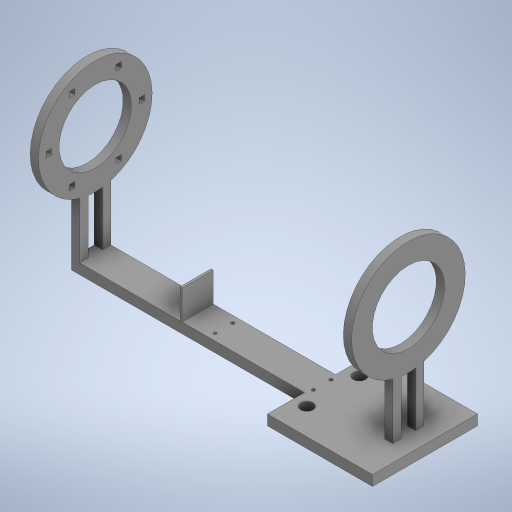
# Autodesk Inventor part: base
Saved by Autodesk Inventor 2023 (Build 270158000, 158)
## iProperties
Created: 2022-11-02
Part Number: base
Material: Generic
Document SubType Name: Modeling
Designer: Admin
Density: 1 g/cm^3
Appearance: Default
Author: Admin
Autodesk Inventor part; units mm, degrees
ref_plane "YZ Plane" through (0, 0, 0) normal (1, 0, 0) x (0, 1, 0)
ref_plane "XZ Plane" through (0, 0, 0) normal (0, 1, 0) x (-1, 0, 0)
ref_plane "XY Plane" through (0, 0, 0) normal (0, 0, 1) x (1, 0, 0)
sketch "Sketch1" plane through (0, 0, 0) normal (1, 0, 0) x (0, 1, 0)
  line L0 (38.9711, 22.5) -> (38.9711, -22.5)
  line L1 (38.9711, -22.5) -> (0, -45)
  line L2 (0, -45) -> (-38.9711, -22.5)
  line L3 (-38.9711, -22.5) -> (-38.9711, 22.5)
  line L4 (-38.9711, 22.5) -> (0, 45)
  line L5 (0, 45) -> (38.9711, 22.5)
  line L6 (0, 45) -> (0, -45)
  line L7 (38.9711, 0) -> (-38.9711, 0)
  circle A0 centre (38.9711, -22.5) radius 17.5
  circle A1 centre (38.9711, -22.5) radius 12.5
  circle A2 centre (38.9711, -22.5) radius 10.4
  circle A3 centre (38.9711, -22.5) radius 15
  line L8 (38.9711, -22.5) -> (62.5188, -22.5)
  line L9 (56.4711, -26.5) -> (64.4711, -26.5)
  line L10 (64.4711, -26.5) -> (64.4711, -18.5)
  line L11 (64.4711, -18.5) -> (56.4711, -18.5)
  line L12 (56.4711, -18.5) -> (56.4711, -26.5)
  line L13 (56.4711, -26.5) -> (64.4711, -18.5) construction
  line L14 (64.4711, -26.5) -> (56.4711, -18.5) construction
  circle A4 centre (38.9711, 22.5) radius 10.4
  circle A5 centre (38.9711, 22.5) radius 12.5
  circle A6 centre (0, 45) radius 10.4
  circle A7 centre (0, 45) radius 12.5
  circle A8 centre (-38.9711, 22.5) radius 10.4
  circle A9 centre (-38.9711, 22.5) radius 12.5
  circle A10 centre (-38.9711, -22.5) radius 10.4
  circle A11 centre (-38.9711, -22.5) radius 12.5
  circle A12 centre (0, -45) radius 10.4
  circle A13 centre (0, -45) radius 12.5
  line L15 (42.9711, 10.6573) -> (42.9711, -10.6573)
  line L16 (34.9711, 10.6573) -> (34.9711, -10.6573)
  line L17 (12.2561, 42.5427) -> (30.715, 31.8855)
  line L18 (8.2561, 35.6145) -> (26.715, 24.9573)
  line L19 (-30.715, 31.8855) -> (-12.2561, 42.5427)
  line L20 (-26.715, 24.9573) -> (-8.2561, 35.6145)
  line L21 (-42.9711, -10.6573) -> (-42.9711, 10.6573)
  line L22 (-34.9711, -10.6573) -> (-34.9711, 10.6573)
  line L23 (-12.2561, -42.5427) -> (-30.715, -31.8855)
  line L24 (-8.2561, -35.6145) -> (-26.715, -24.9573)
  line L25 (30.715, -31.8855) -> (12.2561, -42.5427)
  line L26 (26.715, -24.9573) -> (8.2561, -35.6145)
  line L27 (38.9711, 22.5) -> (0, 0)
  line L28 (29.9645, 17.3) -> (28.1458, 16.25)
  line L29 (-48.9711, -15) -> (-48.9711, 15)
  line L30 (-48.9711, 15) -> (-56.9711, 15)
  line L31 (-56.9711, 15) -> (-56.9711, -15)
  line L32 (-56.9711, -15) -> (-48.9711, -15)
  circle A14 centre (-38.9711, -22.5) radius 17.5
  circle A15 centre (-38.9711, 22.5) radius 17.5
  line L33 (-52.9711, -15) -> (-52.9711, 15)
  line L34 (57.8711, -25.1) -> (63.0711, -25.1)
  line L35 (63.0711, -25.1) -> (63.0711, -19.9)
  line L36 (63.0711, -19.9) -> (57.8711, -19.9)
  line L37 (57.8711, -19.9) -> (57.8711, -25.1)
  line L38 (57.8711, -25.1) -> (63.0711, -19.9) construction
  line L39 (63.0711, -25.1) -> (57.8711, -19.9) construction
  circle A16 centre (38.9711, 22.5) radius 17.5
  circle A17 centre (0, 45) radius 17.5
  circle A18 centre (-38.9711, 22.5) radius 17.5
  circle A19 centre (-38.9711, -22.5) radius 17.5
  circle A20 centre (0, -45) radius 17.5
  line L40 (0, -45) -> (30.2711, -45)
  line L41 (17.5, -49) -> (25.5, -49)
  line L42 (25.5, -49) -> (25.5, -41)
  line L43 (25.5, -41) -> (17.5, -41)
  line L44 (17.5, -41) -> (17.5, -49)
  line L45 (17.5, -49) -> (25.5, -41) construction
  line L46 (25.5, -49) -> (17.5, -41) construction
  line L47 (18.9, -47.6) -> (24.1, -47.6)
  line L48 (24.1, -47.6) -> (24.1, -42.4)
  line L49 (24.1, -42.4) -> (18.9, -42.4)
  line L50 (18.9, -42.4) -> (18.9, -47.6)
  line L51 (18.9, -47.6) -> (24.1, -42.4) construction
  line L52 (24.1, -47.6) -> (18.9, -42.4) construction
  line L53 (-38.9711, -22.5) -> (-4.25, -22.5)
  line L54 (-21.4711, -26.5) -> (-13.4711, -26.5)
  line L55 (-13.4711, -26.5) -> (-13.4711, -18.5)
  line L56 (-13.4711, -18.5) -> (-21.4711, -18.5)
  line L57 (-21.4711, -18.5) -> (-21.4711, -26.5)
  line L58 (-21.4711, -26.5) -> (-13.4711, -18.5) construction
  line L59 (-13.4711, -26.5) -> (-21.4711, -18.5) construction
  line L60 (-20.0711, -25.1) -> (-14.8711, -25.1)
  line L61 (-14.8711, -25.1) -> (-14.8711, -19.9)
  line L62 (-14.8711, -19.9) -> (-20.0711, -19.9)
  line L63 (-20.0711, -19.9) -> (-20.0711, -25.1)
  line L64 (-20.0711, -25.1) -> (-14.8711, -19.9) construction
  line L65 (-14.8711, -25.1) -> (-20.0711, -19.9) construction
  line L66 (56.4711, 26.5) -> (64.4711, 26.5)
  line L67 (64.4711, 26.5) -> (64.4711, 18.5)
  line L68 (64.4711, 18.5) -> (56.4711, 18.5)
  line L69 (56.4711, 18.5) -> (56.4711, 26.5)
  line L70 (56.4711, 26.5) -> (64.4711, 18.5) construction
  line L71 (64.4711, 26.5) -> (56.4711, 18.5) construction
  line L72 (57.8711, 25.1) -> (63.0711, 25.1)
  line L73 (63.0711, 25.1) -> (63.0711, 19.9)
  line L74 (63.0711, 19.9) -> (57.8711, 19.9)
  line L75 (57.8711, 19.9) -> (57.8711, 25.1)
  line L76 (57.8711, 25.1) -> (63.0711, 19.9) construction
  line L77 (63.0711, 25.1) -> (57.8711, 19.9) construction
  line L78 (17.5, 49) -> (25.5, 49)
  line L79 (25.5, 49) -> (25.5, 41)
  line L80 (25.5, 41) -> (17.5, 41)
  line L81 (17.5, 41) -> (17.5, 49)
  line L82 (17.5, 49) -> (25.5, 41) construction
  line L83 (25.5, 49) -> (17.5, 41) construction
  line L84 (18.9, 47.6) -> (24.1, 47.6)
  line L85 (24.1, 47.6) -> (24.1, 42.4)
  line L86 (24.1, 42.4) -> (18.9, 42.4)
  line L87 (18.9, 42.4) -> (18.9, 47.6)
  line L88 (18.9, 47.6) -> (24.1, 42.4) construction
  line L89 (24.1, 47.6) -> (18.9, 42.4) construction
  line L90 (-21.4711, 26.5) -> (-13.4711, 26.5)
  line L91 (-13.4711, 26.5) -> (-13.4711, 18.5)
  line L92 (-13.4711, 18.5) -> (-21.4711, 18.5)
  line L93 (-21.4711, 18.5) -> (-21.4711, 26.5)
  line L94 (-21.4711, 26.5) -> (-13.4711, 18.5) construction
  line L95 (-13.4711, 26.5) -> (-21.4711, 18.5) construction
  line L96 (-20.0711, 25.1) -> (-14.8711, 25.1)
  line L97 (-14.8711, 25.1) -> (-14.8711, 19.9)
  line L98 (-14.8711, 19.9) -> (-20.0711, 19.9)
  line L99 (-20.0711, 19.9) -> (-20.0711, 25.1)
  line L100 (-20.0711, 25.1) -> (-14.8711, 19.9) construction
  line L101 (-14.8711, 25.1) -> (-20.0711, 19.9) construction
  line L102 (0, 0) -> (21.5, 0)
  circle A21 centre (21.5, 0) radius 55
  circle A22 centre (21.5, 0) radius 35
  line L103 (-31.415, 0) -> (-31.415, 15)
  line L104 (-31.415, 15) -> (-85.4711, 15)
  line L105 (-85.4711, 15) -> (-85.4711, 0)
  line L106 (-31.415, 7) -> (-85.4711, 7)
  line L107 (-85.4711, 15) -> (-95.4711, 15)
  line L108 (-95.4711, 15) -> (-95.4711, -10)
  line L109 (-31.415, 0) -> (-31.415, -15)
  line L110 (-31.415, -15) -> (-85.4711, -15)
  line L111 (-85.4711, -15) -> (-85.4711, 0)
  line L112 (-31.415, -7) -> (-85.4711, -7)
  line L113 (-85.4711, -15) -> (-95.4711, -15)
  line L114 (-95.4711, -15) -> (-95.4711, -10)
  point P0 (60.4711, -22.5)
  point P1 (-42.9711, 10.6573)
  point P2 (21.5, -45)
  point P3 (-17.4711, -22.5)
  point P4 (60.4711, 22.5)
  point P5 (21.5, 45)
  point P6 (-17.4711, 22.5)
  point P7 (-31.415, -15)
  point P8 (-31.7663, 15)
  point P9 (-31.2665, 15.5144)
  point P10 (-31.2665, -15.5144)
  point P11 (-31.7663, -15)
  point P12 (-56.9711, 7)
  point P13 (-31.7663, 15)
  point P14 (-46.176, 15)
  point P15 (-56.9711, -7)
  point P16 (-33.0527, 7)
  point P17 (-33.0527, -7)
  point P18 (-28.5742, -22.7504)
  point P19 (-28.5742, 22.7504)
  point P20 (-46.176, -15)
  point P21 (-31.7663, -15)
  dimension "d45" = 110
  dimension "d8" = 35
  dimension "d9" = 45
  dimension "d10" = 25
  dimension "d11" = 20.8
  dimension "d12" = 30
  dimension "d13" = 8
  dimension "d14" = 8
  dimension "d15" = 360
  dimension "d16" = 4
  dimension "d17" = 4
  dimension "d18" = 360
  dimension "d22" = 30
  dimension "d23" = 8
  dimension "d24" = 30
  dimension "d25" = 35
  dimension "d26" = 35
  dimension "d27" = 4
  dimension "d30" = 5.2
  dimension "d31" = 5.2
  dimension "d34" = 360
  dimension "d36" = 8
  dimension "d37" = 8
  dimension "d38" = 5.2
  dimension "d39" = 5.2
  dimension "d40" = 8
  dimension "d41" = 8
  dimension "d42" = 5.2
  dimension "d43" = 5.2
  dimension "d44" = 21.5
  dimension "d46" = 70
  dimension "d47" = 15
  dimension "d49" = 8
  dimension "d50" = 28.5
  dimension "d51" = 10
  constraints: 230 end point, 32 symmetric about line, 20 centre point, 16 midpoint, 14 coincident, 12 horizontal, 11 parallel, 11 perpendicular, 11 point on line, 7 point on circle, 4 vertical, 3 tangent, 97 other
  measures "d8" diameter of A0
  measures "d9" distance of L0.start L0.end
  measures "d10" diameter of A1
  measures "d11" diameter of A2
  measures "d12" diameter of A3
  measures "d13" distance of L11.end L10.end
  measures "d14" distance of L9.end L10.end
  measures "d16" distance between parallel lines of L15 L0
  measures "d17" distance between parallel lines of L0 L16
  measures "d22" distance of L29.start L29.end
  measures "d23" distance of L30.start L30.end
  measures "d24" distance of L30.end L31.end
  measures "d25" diameter of A14
  measures "d26" diameter of A15
  measures "d27" distance between parallel lines of L31 L33
  measures "d30" distance of L36.end L35.end
  measures "d31" distance of L34.end L35.end
  measures "d36" distance of L43.end L42.end
  measures "d37" distance of L41.end L42.end
  measures "d38" distance of L49.end L48.end
  measures "d39" distance of L47.end L48.end
  measures "d40" distance of L56.end L55.end
  measures "d41" distance of L54.end L55.end
  measures "d42" distance of L62.end L61.end
  measures "d43" distance of L60.end L61.end
  measures "d44" distance of L27.end L102.end
  measures "d46" diameter of A22
  measures "d47" distance of L103.start L103.end
  measures "d49" distance between parallel lines of L104 L106
  measures "d50" distance between parallel lines of L31 L105
  measures "d51" distance of L104.end L107.end
extrude "Extrusion1" add sketch "Sketch1" along normal blind 8 contours L5 A4 A22 L0 | L27 A4 L5 | L0 A4 L27 | A4 A22 A5 L0 | L0 A5 L27 A4 | A4 L27 A5 L5 | L5 A5 A22 A4 | A5 L15 A16 L0 | L0 A16 L16 A5 | A22 A4 | A4 A22 A5 | A5 L18 A16 L5 | L5 A16 L17 A5 | L27 A16 L18 A5 | A5 L16 A16 L27 | A16 L15 A0 L0 | L0 L7 L16 A16 | A5 A22 A16 L15 | A5 A22 A16 | A16 L18 A17 A22 L5 | L5 A22 L17 A16 | L17 A16 A22 A5 | A16 L16 L7 L27 | L27 L6 A17 L18 A16 | L0 A0 L16 L7 | A16 A22 A0 L15 | L12 L11 L10 L9 | L44 L43 L42 L40 L48 L49 L50 | L40 L50 L47 L48 L42 L41 L44 | L81 L78 L79 L80 | L69 L66 L67 L68 | A16 A22 L17 A17 A21 A20 L25 A0 | A22 A17 L5 | L5 A17 L17 A22 | L17 A22 A16 | L7 A22 A17 L6 | L7 L16 A0 L26 A20 L6 | L6 A20 A22 L7 | A0 L15 A3 L0 | L0 A3 L16 A0 | A0 A22 A3 L15 | A17 A22 L18 A7 L5 | L5 A7 L17 A17 | A17 L18 A22 | A17 L6 A22 L18 | A17 A22 L6 | A20 L26 A22 L6 | L6 A22 A20 | A22 L53 L55 L56 L57 A14 L109 L7 | L93 L90 L91 L92 | L7 L103 A15 L20 A17 A22 | A3 L15 A1 L0 | L0 A1 L16 A3 | L16 A3 L26 A0 | A0 L8 A3 A22 | A3 A22 A1 L15 | A7 L6 A6 L5 | L5 A6 A21 A7 | L17 A7 A21 A17 | A22 L6 A7 L18 | A22 A17 L20 A7 L6 | A22 L26 A13 L6 | L6 A13 L24 A20 A22 | A20 A22 L26 | L26 A0 L1 A22 A20 | A20 L24 A14 L57 L54 L55 L53 A22 | L109 A14 A21 L7 | L7 A21 A15 L103 | A1 A22 A2 L0 | L0 A2 L1 A1 | L16 A1 L26 A3 | L26 A3 L1 A0 | A0 A22 A3 L8 | A3 L8 A1 A22 | A6 L6 L5 | L5 L4 A6 A21 | A7 L4 A6 L6 | A17 L4 A7 L20 | L20 A15 A21 L4 A17 | A13 L1 A12 L6 | L6 A12 L2 A13 | A22 A20 L1 A13 L26 | A22 L1 A20 | A20 L2 A21 A14 L24 | L24 A13 L2 A20 | L103 A9 L20 A15 | A15 A21 L106 L103 | L109 L112 A21 A14 | A14 L53 A11 L109 | L55 L54 L57 L53 L63 L60 L61 | L53 L61 L62 L63 L57 L56 L55 | A2 A22 L8 L0 | L0 L1 A2 | L26 A1 L1 A3 | A0 L25 A22 L1 | L1 A3 L25 A0 | A22 L25 A0 | A0 L25 A3 A22 | A3 A22 A1 L8 | A1 L8 A2 A22 | L6 A6 L4 | L20 A9 A21 A15 | A17 A21 L19 A7 L4 | L4 A21 A17 | A12 L1 L6 | L6 L2 A12 | A20 L25 A13 L1 | L1 A22 L25 A20 | A14 A21 A11 L24 | L24 A11 L53 A14 | A20 A21 L2 | L2 A13 L23 A21 A20 | L106 A21 A9 L103 | L109 A11 A21 L112 | L61 L60 L63 L53 | L53 L63 L62 L61 | L8 A22 A2 L1 | A2 L8 A22 | A2 A22 A1 L1 | L1 A1 L25 A3 | A3 L25 A1 A22 | A1 A22 A2 L8 | L4 A7 A21 A6 | A9 L103 A21 A8 | L40 A12 A21 L2 | L1 A12 L40 | L1 A13 L40 A12 | A12 A21 A13 L2 | A20 L40 A13 L25 | A11 A21 A10 L53 | L106 L22 A9 A21 | A21 A11 L22 L112 | A9 A21 L103 | L53 A10 A21 L109 A11 | L109 A21 A11 | L8 A2 A22 | A7 L19 A21 | A21 A13 L40 A20 | L40 A13 A21 A12 | A13 A21 L23 | L22 A11 L3 L112 | L106 L3 A9 L22 | A9 L3 A8 L104 A21 | A21 L110 A10 L3 A11 | L53 A21 A10 | A10 A21 L53 | A15 L33 L106 L31 L30 | L30 L33 A15 | A8 A21 | L50 L49 L48 L40 | L40 L48 L47 L50 | L3 A11 L21 L112 | L106 L21 A9 L3 | A8 L3 L104 | L110 L3 A10 | L104 A8 L3 A9 | A9 L21 L106 A15 L29 | L29 A15 L33 L30 | L31 L106 L105 L104 | A15 L29 L106 L33 | A14 L33 L32 | L32 L31 L112 L33 A14 | L3 A10 L110 A11 | L21 A11 L29 A14 L112 | A14 L29 L112 | L106 L29 A15 | A8 L104 L3 | L3 L110 A10 | L105 L111 L113 L114 L108 L107 | L32 L33 A14 L29 | L110 L111 L112 L31 | L33 L112 L29 A14 | L37 L36 L35 L34 | L72 L73 L74 L75 | L84 L85 L86 L87 | L96 L97 L98 L99
extrude "Extrusion2" cut sketch "Sketch1" along normal blind 8 contours L5 A4 A22 L0 | L27 A4 L5 | L0 A4 L27 | A4 A22 A5 L0 | L0 A5 L27 A4 | A4 L27 A5 L5 | L5 A5 A22 A4 | A5 L15 A16 L0 | L0 A16 L16 A5 | A5 L18 A16 L5 | L5 A16 L17 A5 | L27 A16 L18 A5 | A5 L16 A16 L27 | A16 L15 A0 L0 | L0 L7 L16 A16 | A5 A22 A16 L15 | A16 L18 A17 A22 L5 | L5 A22 L17 A16 | L17 A16 A22 A5 | A16 L16 L7 L27 | L27 L6 A17 L18 A16 | L0 A0 L16 L7 | A16 A22 A0 L15 | L17 A22 A16 | L7 A22 A17 L6 | L7 L16 A0 L26 A20 L6 | L6 A20 A22 L7 | A0 L15 A3 L0 | L0 A3 L16 A0 | A0 A22 A3 L15 | A17 L18 A22 | A17 L6 A22 L18 | A17 A22 L6 | A20 L26 A22 L6 | L6 A22 A20 | A3 L15 A1 L0 | L0 A1 L16 A3 | L16 A3 L26 A0 | A3 A22 A1 L15 | A20 A22 L26 | L26 A0 L1 A22 A20 | A1 A22 A2 L0 | L0 A2 L1 A1 | L16 A1 L26 A3 | L26 A3 L1 A0 | A2 A22 L8 L0 | L0 L1 A2 | L26 A1 L1 A3 | A0 L25 A22 L1 | L1 A3 L25 A0 | A22 L25 A0 | A0 L25 A3 A22 | L61 L60 L63 L53 | L53 L63 L62 L61 | L8 A22 A2 L1 | A2 A22 A1 L1 | L1 A1 L25 A3 | A3 L25 A1 A22 | L50 L49 L48 L40 | L40 L48 L47 L50 | L37 L36 L35 L34 | L72 L73 L74 L75 | L84 L85 L86 L87 | L96 L97 L98 L99
extrude "Extrusion3" add sketch "Sketch1" along normal blind 327 contours L105 L111 L113 L114 L108 L107
sketch "Sketch2" plane through (0, -95.4711, -15) normal (0, -1, 0) x (1, 0, 0)
  line L0 (327, 0) -> (327, 30) projected
  line L1 (327, 15) -> (239.7614, 15)
  line L2 (225.4, -35.8) -> (327, -35.8)
  line L3 (327, -35.8) -> (327, 65.8)
  line L4 (327, 65.8) -> (225.4, 65.8)
  line L5 (225.4, 65.8) -> (225.4, -35.8)
  line L6 (225.4, -35.8) -> (327, 65.8) construction
  line L7 (327, -35.8) -> (225.4, 65.8) construction
  line L8 (327, 30) -> (327, 0) projected
  circle A0 centre (238.1, -10.4) radius 6
  circle A1 centre (301.9, 15) radius 3.25
  line L9 (8, -40) -> (8, 70) projected
  line L10 (8, 50) -> (8, -20) projected
  line L11 (8, 15) -> (107, 15)
  line L12 (107, 15) -> (132.5, 15)
  line L13 (132.5, 15) -> (132.5, 6.5)
  circle A2 centre (132.5, 6.5) radius 1.5
  circle A3 centre (132.5, 23.5) radius 1.5
  circle A4 centre (227.5, 6.5) radius 1.5
  circle A5 centre (227.5, 23.5) radius 1.5
  circle A6 centre (238.1, 40.4) radius 6
  line L14 (107, 0) -> (105, 0)
  line L15 (105, 0) -> (105, 30)
  line L16 (105, 30) -> (107, 30)
  line L17 (107, 30) -> (107, 0)
  point P0 (0, 15)
  point P1 (276.2, 15)
  point P2 (8, 0)
  point P3 (8, 30)
  dimension "d58" = 101.6
  dimension "d59" = 101.6
  dimension "d60" = 12
  dimension "d63" = 6.5
  dimension "d65" = 99
  dimension "d66" = 25.5
  dimension "d67" = 8.5
  dimension "d68" = 3
  dimension "d71" = 95
  dimension "d80" = 25.4
  dimension "d81" = 12.7
  dimension "d82" = 76.5
  dimension "d92" = 2
  constraints: 28 end point, 7 centre point, 6 horizontal, 5 midpoint, 4 parallel, 3 perpendicular, 2 point on line, 2 symmetric about line, 1 coincident, 1 collinear, 6 other
  measures "d58" distance of L4.end L3.end
  measures "d59" distance of L2.end L3.end
  measures "d60" diameter of A0
  measures "d63" diameter of A1
  measures "d65" distance of L11.start L11.end
  measures "d66" distance of L11.end L12.end
  measures "d67" distance of L12.end L13.end
  measures "d68" diameter of A2
  measures "d71" distance of A2.centre A4.centre
  measures "d80" distance from line of L2 A0.centre
  measures "d81" distance from line of L5 A0.centre
  measures "d82" distance from line of L5 A1.centre
  measures "d92" distance between parallel lines of L15 L17
extrude "Extrusion4" add sketch "Sketch2" against normal blind 10 contours L3 L2 L5 L4 L0
extrude "Extrusion5" cut sketch "Sketch2" against normal blind 10 contours A2 | A3 | A4 | A5
pattern_linear "Rectangular Pattern1" count 2 spacing 303 along (1, 0, 0) of "Extrusion1", "Extrusion2"
sketch "Sketch3" plane through (0, 0, 0) normal (-1, 0, 0) x (0, 0, 1)
  line L0 (15, -31.415) -> (15, -95.4711) projected
  arc A0 (15, -31.415) -> (-15, -31.415) centre (0, 21.5) ccw projected
  line L1 (-15, -95.4711) -> (-15, -31.415) projected
  line L2 (15, -95.4711) -> (-15, -95.4711) projected
  line L3 (-7, -85.4711) -> (7, -85.4711) projected
  line L4 (-7, -33.0527) -> (-7, -85.4711) projected
  arc A1 (-7, -33.0527) -> (7, -33.0527) centre (0, 21.5) ccw projected
  line L5 (7, -85.4711) -> (7, -33.0527) projected
  circle A2 centre (0, 21.5) radius 35 projected
  line L6 (-25.1, -20.0711) -> (-25.1, -14.8711) projected
  line L7 (-25.1, -14.8711) -> (-19.9, -14.8711) projected
  line L8 (-19.9, -14.8711) -> (-19.9, -20.0711) projected
  line L9 (-19.9, -20.0711) -> (-25.1, -20.0711) projected
  line L10 (-42.4, 24.1) -> (-42.4, 18.9) projected
  line L11 (-42.4, 18.9) -> (-47.6, 18.9) projected
  line L12 (-47.6, 18.9) -> (-47.6, 24.1) projected
  line L13 (-47.6, 24.1) -> (-42.4, 24.1) projected
  line L14 (25.1, 63.0711) -> (25.1, 57.8711) projected
  line L15 (25.1, 57.8711) -> (19.9, 57.8711) projected
  line L16 (19.9, 57.8711) -> (19.9, 63.0711) projected
  line L17 (19.9, 63.0711) -> (25.1, 63.0711) projected
  line L18 (25.1, -20.0711) -> (19.9, -20.0711) projected
  line L19 (19.9, -20.0711) -> (19.9, -14.8711) projected
  line L20 (19.9, -14.8711) -> (25.1, -14.8711) projected
  line L21 (25.1, -14.8711) -> (25.1, -20.0711) projected
  line L22 (-19.9, 63.0711) -> (-19.9, 57.8711) projected
  line L23 (-19.9, 57.8711) -> (-25.1, 57.8711) projected
  line L24 (-25.1, 57.8711) -> (-25.1, 63.0711) projected
  line L25 (-25.1, 63.0711) -> (-19.9, 63.0711) projected
  line L26 (47.6, 18.9) -> (42.4, 18.9) projected
  line L27 (42.4, 18.9) -> (42.4, 24.1) projected
  line L28 (42.4, 24.1) -> (47.6, 24.1) projected
  line L29 (47.6, 24.1) -> (47.6, 18.9) projected
  point P0 (0, 0)
extrude "Extrusion7" add sketch "Sketch3" against normal blind 3.1 contours L6 L7 L8 L9 | L10 L11 L12 L13 | L14 L15 L16 L17 | L18 L19 L20 L21 | L22 L23 L24 L25 | L26 L27 L28 L29
sketch "Sketch4" plane through (311, -85.4711, -15) normal (1, 0, 0) x (0, 0, -1)
  line L0 (-57.4, 104.3711) -> (-62.6, 104.3711) projected
  line L1 (-62.6, 104.3711) -> (-62.6, 109.5711) projected
  line L2 (-62.6, 109.5711) -> (-57.4, 109.5711) projected
  line L3 (-57.4, 109.5711) -> (-57.4, 104.3711) projected
  line L4 (4.9, 143.3423) -> (4.9, 148.5423) projected
  line L5 (4.9, 148.5423) -> (10.1, 148.5423) projected
  line L6 (10.1, 148.5423) -> (10.1, 143.3423) projected
  line L7 (10.1, 143.3423) -> (4.9, 143.3423) projected
  line L8 (-34.9, 65.4) -> (-40.1, 65.4) projected
  line L9 (-40.1, 65.4) -> (-40.1, 70.6) projected
  line L10 (-40.1, 70.6) -> (-34.9, 70.6) projected
  line L11 (-34.9, 70.6) -> (-34.9, 65.4) projected
  line L12 (-40.1, 143.3423) -> (-40.1, 148.5423) projected
  line L13 (-40.1, 148.5423) -> (-34.9, 148.5423) projected
  line L14 (-34.9, 148.5423) -> (-34.9, 143.3423) projected
  line L15 (-34.9, 143.3423) -> (-40.1, 143.3423) projected
  line L16 (27.4, 104.3711) -> (27.4, 109.5711) projected
  line L17 (27.4, 109.5711) -> (32.6, 109.5711) projected
  line L18 (32.6, 109.5711) -> (32.6, 104.3711) projected
  line L19 (32.6, 104.3711) -> (27.4, 104.3711) projected
  line L20 (10.1, 70.6) -> (10.1, 65.4) projected
  line L21 (10.1, 65.4) -> (4.9, 65.4) projected
  line L22 (4.9, 65.4) -> (4.9, 70.6) projected
  line L23 (4.9, 70.6) -> (10.1, 70.6) projected
  circle A0 centre (-15, 106.9711) radius 35 projected
  line L24 (0, 0) -> (-8, 0) projected
  line L25 (0, 0) -> (0, 54.0561) projected
  arc A1 (0, 54.0561) -> (-30, 54.0561) centre (-15, 106.9711) ccw projected
  line L26 (-30, 54.0561) -> (-30, 0) projected
  line L27 (-22, 0) -> (-30, 0) projected
  line L28 (-22, 0) -> (-22, 52.4184) projected
  arc A2 (-22, 52.4184) -> (-8, 52.4184) centre (-15, 106.9711) ccw projected
  line L29 (-8, 52.4184) -> (-8, 0) projected
  point P0 (-15, 85.4711)
extrude "Extrusion8" add sketch "Sketch4" against normal blind 3.1 contours L0 L1 L2 L3 | L4 L5 L6 L7 | L8 L9 L10 L11 | L12 L13 L14 L15 | L16 L17 L18 L19 | L20 L21 L22 L23
extrude "Extrusion9" add sketch "Sketch2" against normal blind 38.5 contours L15 L16 L17 L11 | L11 L17 L14 L15
equation "\"d14\" = d13"
equation "\"d17\" = d16"
equation "\"d31\" = d30"
equation "\"d37\" = d36"
equation "\"d39\" = d38"
equation "\"d41\" = d40"
equation "\"d43\" = d42"
body "Solid1"
